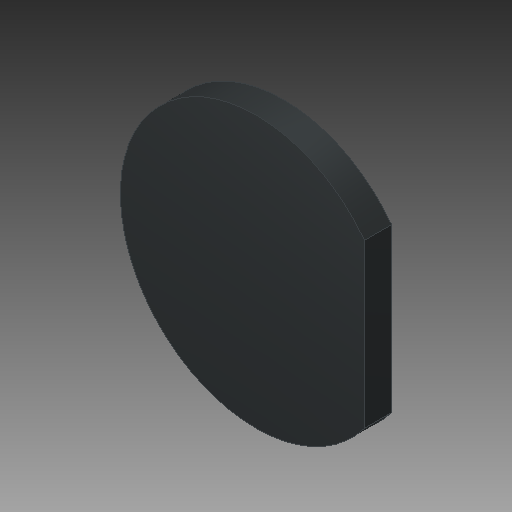
# Autodesk Inventor part: Flywheel
Saved by Autodesk Inventor 2019 (Build 230136000, 136)
## iProperties
Created: 2019-08-25
Part Number: Flywheel
Material: Iron, Cast
Document SubType Name: Modeling
Designer: DIBYOJYOTI
Density: 7.15 g/cm^3
Appearance: Iron Gray
Mass: 66.5417 g
Surface Area: 44.9714 cm^2
Volume: 9.30654 cm^3
Author: DIBYOJYOTI
Autodesk Inventor part; units mm, degrees
ref_plane "YZ Plane" through (0, 0, 0) normal (1, 0, 0) x (0, 1, 0)
ref_plane "XZ Plane" through (0, 0, 0) normal (0, 1, 0) x (-1, 0, 0)
ref_plane "XY Plane" through (0, 0, 0) normal (0, 0, 1) x (1, 0, 0)
sketch "Sketch1" plane through (0, 0, 0) normal (0, 0, 1) x (1, 0, 0)
  arc A0 (20, 15) -> (20, -15) centre (0, 0) ccw
  line L0 (20, 0) -> (20, -15)
  line L1 (20, 0) -> (20, 15)
  circle A1 centre (0, 0) radius 2
  dimension "d0" = 50
  dimension "d3" = 4
  constraints: 4 end point, 2 centre point, 2 coincident, 2 point on circle, 1 point on line, 1 vertical
  measures "d0" diameter of A0
  measures "d3" diameter of A1
extrude "Extrusion1" add sketch "Sketch1" along normal blind 5 contours L1 L0 A0 | A1
body "Solid1"
